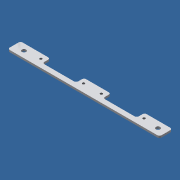
# Autodesk Inventor part: DriverMount
Saved by Autodesk Inventor 2016 (Build 200138000, 138)
## iProperties
Created: 2016-03-04
Part Number: DriverMount
Material: Aluminium 6061
Document SubType Name: Modeling
Designer: 4ndreas
Density: 2.7 g/cm^3
Appearance: Aluminium - flach
Mass: 7.67265 g
Surface Area: 36.717 cm^2
Volume: 2.84172 cm^3
Author: 4ndreas
Autodesk Inventor part; units mm, degrees
ref_plane "YZ Plane" through (0, 0, 0) normal (1, 0, 0) x (0, 1, 0)
ref_plane "XZ Plane" through (0, 0, 0) normal (0, 1, 0) x (-1, 0, 0)
ref_plane "XY Plane" through (0, 0, 0) normal (0, 0, 1) x (1, 0, 0)
sketch "Skizze1" plane through (0, 0, 0) normal (0, 0, 1) x (1, 0, 0)
  circle A0 centre (2.5, 77) radius 1.875 construction
  circle A1 centre (45.5, 77) radius 1.875 construction
  circle A2 centre (2.5, 8) radius 1.875 construction
  circle A3 centre (45.5, 8) radius 1.875 construction
  line L0 (-1, 5) -> (-1, 80) construction
  line L1 (49, 5) -> (-1, 5) construction
  line L2 (49, 80) -> (49, 5) construction
  line L3 (-1, 80) -> (49, 80) construction
  circle A4 centre (63.5, 77) radius 1.875 construction
  circle A5 centre (106.5, 77) radius 1.875 construction
  circle A6 centre (63.5, 8) radius 1.875 construction
  circle A7 centre (106.5, 8) radius 1.875 construction
  line L4 (60, 5) -> (60, 80) construction
  line L5 (110, 5) -> (60, 5) construction
  line L6 (110, 80) -> (110, 5) construction
  line L7 (60, 80) -> (110, 80) construction
  line L8 (-3, 0) -> (-3, 85) construction
  line L9 (-23, 0) -> (-23, 85) construction
  line L10 (-16.375, 0) -> (-21, 0) construction
  line L11 (-23, 0) -> (-21, 0) construction
  line L12 (-16.375, 0) -> (-15.575, 0) construction
  line L13 (0, 0) -> (-9.625, 0) construction
  line L14 (118.625, 85) -> (114, 85) construction
  line L15 (114, 0) -> (114, 85) construction
  line L16 (118.625, 0) -> (114, 0) construction
  line L17 (118.625, 0) -> (118.625, 85) construction
  line L18 (112, 0) -> (114, 0) construction
  line L19 (112, 0) -> (112, 85) construction
  line L20 (132, 0) -> (132, 85) construction
  line L21 (130, 0) -> (132, 0) construction
  line L22 (-23, 0) -> (132, 0)
  line L23 (132, 0) -> (132, 5)
  line L24 (132, 5) -> (-23, 5)
  line L25 (-23, 5) -> (-23, 0)
  line L26 (102, 13) -> (132, 13)
  line L27 (132, 13) -> (132, 5)
  line L28 (132, 5) -> (102, 5)
  line L29 (102, 5) -> (102, 13)
  line L30 (41, 5) -> (68, 5)
  line L31 (68, 5) -> (68, 13)
  line L32 (68, 13) -> (41, 13)
  line L33 (41, 13) -> (41, 5)
  line L34 (-23, 5) -> (7, 5)
  line L35 (7, 5) -> (7, 13)
  line L36 (7, 13) -> (-23, 13)
  line L37 (-23, 13) -> (-23, 5)
  line L38 (49, 5) -> (60, 5) construction
  line L39 (54.5, 0.9478) -> (54.5, 9.0522) construction
  line L40 (130, 0) -> (114, 0) construction
  line L41 (114, 0) -> (114, 13) construction
  line L42 (114, 13) -> (130, 13) construction
  line L43 (130, 13) -> (130, 0) construction
  line L44 (130, 0) -> (114, 13) construction
  line L45 (114, 0) -> (130, 13) construction
  line L46 (-23, 0) -> (-3, 0) construction
  line L47 (-3, 0) -> (-3, 13) construction
  line L48 (-3, 13) -> (-23, 13) construction
  line L49 (-23, 13) -> (-23, 0) construction
  line L50 (-23, 0) -> (-3, 13) construction
  line L51 (-3, 0) -> (-23, 13) construction
  point P0 (54.5, 5)
  point P1 (122, 6.5)
  point P2 (-13, 6.5)
  dimension "d0" = 8
  dimension "d1" = 8
  dimension "d2" = 8
  constraints: 60 end point, 12 parallel, 7 perpendicular, 6 collinear, 6 horizontal, 6 midpoint, 5 point on line, 1 vertical, 2 other
  measures "d0" distance between parallel lines of L35 L0
  measures "d1" distance between parallel lines of L2 L33
  measures "d2" distance between parallel lines of L24 L36
extrude "Extrusion1" add sketch "Skizze1" along normal blind 2
sketch "Skizze2" plane through (0, 0, 0) normal (0, 0, -1) x (-1, 0, 0)
  point P0 (0, 0)
  point P1 (-106.5, 8)
  point P2 (-63.5, 8)
  point P3 (-45.5, 8)
  point P4 (-2.5, 8)
hole "Bohrung1" at (106.5, 8, 0) at (63.5, 8, 0) at (45.5, 8, 0) at (2.5, 8, 0) direction (0, 0, 1) diameter 2.459 end through all thread size "M3x0.5" class "6H" standard "ANSI Metric M Profile"
fillet "Rundung1" radius 2 12 edges at (102, 5, 1) (102, 13, 1) (68, 5, 1) (68, 13, 1) (41, 13, 1) (41, 5, 1) (7, 5, 1) (7, 13, 1) (-23, 13, 1) (-23, 0, 1) (132, 0, 1) (132, 13, 1)
sketch "Skizze3" plane through (0, 0, 0) normal (0, 0, -1) x (-1, 0, 0)
  point P0 (0, 0)
  point P1 (13, 6.5)
  point P2 (-122, 6.5)
hole "Bohrung2" at (-13, 6.5, 0) at (122, 6.5, 0) direction (0, 0, 1) diameter 4.2 end through all
